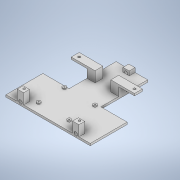
# Autodesk Inventor part: Electronics_holder
Saved by Autodesk Inventor 2020 (Build 240168000, 168)
## iProperties
Created: 2020-06-07
Part Number: Electronics_holder
Material: Generic
Document SubType Name: Modeling
Designer: Abhinav Roy
Density: 1 g/cm^3
Appearance: Default
Author: Abhinav Roy
Autodesk Inventor part; units mm, degrees
ref_plane "YZ Plane" through (0, 0, 0) normal (1, 0, 0) x (0, 1, 0)
ref_plane "XZ Plane" through (0, 0, 0) normal (0, 1, 0) x (-1, 0, 0)
ref_plane "XY Plane" through (0, 0, 0) normal (0, 0, 1) x (1, 0, 0)
sketch "Sketch1" plane through (0, 0, 0) normal (0, 1, 0) x (-1, 0, 0)
  line L0 (0, 0) -> (-30, 0)
  line L1 (-30, 0) -> (-30, -159)
  line L2 (-30, -159) -> (0, -159)
  line L3 (0, -159) -> (0, 0)
  line L4 (0, 0) -> (50, 0)
  line L5 (50, 0) -> (50, -70)
  line L6 (50, -70) -> (0, -70)
  line L7 (0, -70) -> (0, 0)
  dimension "d0" = 159
  dimension "d1" = 30
  dimension "d2" = 50
  dimension "d3" = 70
  constraints: 16 end point, 4 parallel, 2 horizontal, 2 perpendicular
  measures "d0" distance of L2.end L0.start
  measures "d1" distance of L0.start L0.end
  measures "d2" distance of L5.end L6.end
  measures "d3" distance of L4.end L5.end
extrude "Extrusion1" add sketch "Sketch1" along normal blind 4
sketch "Sketch2" plane through (0, 4, 0) normal (0, 1, 0) x (1, 0, 0)
  line L0 (-16.5, 0) -> (-16.5, 11)
  line L1 (-16.5, 11) -> (-28.5, 11)
  line L2 (30, 159) -> (0, 159) projected
  line L3 (30, 159) -> (24, 159)
  line L4 (24, 159) -> (24, 148)
  line L5 (24, 148) -> (30, 148)
  line L6 (30, 148) -> (30, 159)
  line L7 (-28.5, 11) -> (-28.5, 0)
  line L8 (-50, 0) -> (30, 0) projected
  line L9 (-16.5, 0) -> (-28.5, 0)
  line L10 (-50, 70) -> (-50, 0) projected
  line L11 (30, 0) -> (30, 159) projected
  point P0 (0, 0)
  dimension "d6" = 12
  dimension "d7" = 11
  dimension "d8" = 6
  dimension "d52" = 46.5
  constraints: 16 end point, 5 parallel, 2 perpendicular, 1 horizontal, 1 point on line, 1 vertical
  measures "d6" distance of L0.end L1.end
  measures "d7" distance of L0.start L0.end
  measures "d8" distance of L4.end L5.end
  measures "d52" distance between parallel lines of L11 L0
extrude "Extrusion2" add sketch "Sketch2" along normal blind 8 contours L6 L5 L4 L2
extrude "Extrusion4" add sketch "Sketch2" along normal blind 20 contours L8 L7 L1 L0
sketch "Sketch9" plane through (0, 4, 0) normal (0, 1, 0) x (1, 0, 0)
  line L0 (30, 0) -> (30, 148) construction
  line L1 (30, 111.5) -> (0, 111.5) construction
  line L2 (-16.5, 0) -> (30, 0) construction
  line L3 (0, 159) -> (0, 70) projected
  line L4 (15, 119) -> (0, 119)
  line L5 (0, 119) -> (0, 104) construction
  line L6 (0, 104) -> (15, 104)
  line L7 (15, 104) -> (15, 119)
  line L8 (15, 119) -> (0, 104) construction
  line L9 (0, 119) -> (15, 104) construction
  point P0 (0, 0)
  point P1 (7.5, 111.5)
  point P2 (0, 119)
  dimension "d63" = 111.5
  dimension "d64" = 15
  dimension "d65" = 15
  constraints: 14 end point, 3 point on line, 2 horizontal, 2 midpoint, 2 parallel, 1 perpendicular
  measures "d63" distance between parallel lines of L1 L2
  measures "d64" distance of L5.end L6.end
  measures "d65" distance of L6.end L4.start
extrude "Extrusion5" add sketch "Sketch9" along normal blind 20
sketch "Sketch10" plane through (0, 0, -159) normal (-1, 0, 0) x (0, 0, 1)
  line L0 (40, 24) -> (55, 24) projected
  line L1 (40, 24) -> (55, 24)
  line L2 (55, 24) -> (55, 20)
  line L3 (55, 20) -> (40, 20)
  line L4 (40, 20) -> (40, 24)
  point P0 (159, 0)
  dimension "d68" = 4
  constraints: 8 end point, 2 parallel, 1 horizontal, 1 perpendicular
  measures "d68" distance of L1.end L2.end
extrude "Extrusion6" add sketch "Sketch10" along normal blind 30
sketch "Sketch11" plane through (0, 24, 0) normal (0, 1, 0) x (1, 0, 0)
  line L0 (-30, 104) -> (-30, 119) projected
  line L1 (15, 104) -> (-30, 104) projected
  point P0 (0, 0)
  point P1 (-22.5, 111.5)
  dimension "d71" = 7.5
  dimension "d82" = 7.5
  measures "d71" distance from line of L0 point (-22.5, 111.5)
  measures "d82" distance from line of L1 point (-22.5, 111.5)
hole "Hole5" at (-22.5, 24, -111.5) direction (0, -1, 0) diameter 4.6 depth 6
mirror "Mirror1" about plane through (30, 0, 0) normal (1, 0, 0) of "Extrusion1", "Extrusion2", "Extrusion4", "Extrusion5", "Hole5", "Extrusion6"
sketch "Sketch5" plane through (0, 4, 0) normal (0, 1, 0) x (1, 0, 0)
  line L0 (-50, 0) -> (110, 0) construction
  line L1 (30, 0) -> (30, 159)
  line L2 (0, 159) -> (60, 159) projected
  line L3 (-5.5, 66.5) -> (52.5, 66.5) construction
  line L4 (52.5, 66.5) -> (52.5, 17.5) construction
  line L5 (52.5, 17.5) -> (-5.5, 17.5) construction
  line L6 (-5.5, 17.5) -> (-5.5, 66.5) construction
  line L7 (-5.5, 66.5) -> (52.5, 17.5) construction
  line L8 (52.5, 66.5) -> (-5.5, 17.5) construction
  circle A0 centre (52.5, 17.5) radius 3.5
  circle A1 centre (-5.5, 17.5) radius 3.5
  circle A2 centre (-5.5, 66.5) radius 3.5
  circle A3 centre (52.5, 66.5) radius 3.5
  point P0 (-13, 0)
  point P1 (73, 0)
  point P2 (23.5, 42)
  dimension "d31" = 58
  dimension "d32" = 49
  dimension "d33" = 7
  dimension "d45" = 42
  dimension "d79" = 13
  constraints: 14 end point, 4 centre point, 4 coincident, 4 midpoint, 3 equal radius, 2 parallel, 1 horizontal, 1 perpendicular
  measures "d31" distance of L4.end L5.end
  measures "d32" distance of L3.end L4.end
  measures "d33" diameter of A0
  measures "d45" distance from line of L0 point (23.5, 42)
  measures "d79" diameter of point (23.5, 42) L1
extrude "Extrusion3" add sketch "Sketch5" along normal blind 2
sketch "Sketch6" plane through (52.5, 6, -17.5) normal (0, 1, 0) x (1, 0, 0)
  circle A0 centre (-58, 0) radius 3.5 construction
  circle A1 centre (-58, 49) radius 3.5 construction
  circle A2 centre (0, 49) radius 3.5 construction
  point P0 (-52.5, -17.5)
  point P1 (0, 0)
  point P2 (-58, 0)
  point P3 (-58, 49)
  constraints: 3 coincident
hole "Hole3" at (52.5, 6, -66.5) at (52.5, 6, -17.5) at (-5.5, 6, -17.5) at (-5.5, 6, -66.5) direction (0, -1, 0) diameter 1.8 depth 6
sketch "Sketch4" plane through (-50, 12, 0) normal (0, 0, 1) x (1, 0, 0)
  line L0 (0, -12) -> (0, -8) projected
  line L1 (0, -12) -> (160, -12) projected
  line L2 (160, -12) -> (160, -8) projected
  line L3 (21.5, -8) -> (21.5, 12) projected
  line L4 (126.5, -8) -> (126.5, 12) projected
  point P0 (50, -12)
  point P1 (27.5, -6)
  point P2 (132.5, -6)
  point P3 (160, 0)
  dimension "d21" = 6
  dimension "d22" = 6
  dimension "d53" = 6
  dimension "d54" = 6
  measures "d21" distance from line of L1 point (27.5, -6)
  measures "d22" distance from line of L1 point (132.5, -6)
  measures "d53" distance from line of L3 point (27.5, -6)
  measures "d54" distance from line of L4 point (132.5, -6)
hole "Hole2" at (-22.5, 6, 0) at (82.5, 6, 0) direction (0, 0, -1) diameter 5.9 depth 11 countersink diameter 6.8 countersink angle 45
sketch "Sketch3" plane through (0, 0, -159) normal (0, 0, -1) x (-1, 0, 0)
  line L0 (-24, 12) -> (-36, 12) projected
  line L1 (-36, 4) -> (-36, 12) projected
  point P0 (0, 0)
  point P1 (-30, 6)
  dimension "d11" = 6
  dimension "d12" = 6
  measures "d11" distance from line of L0 point (-30, 6)
  measures "d12" distance from line of point (-30, 6) L1
hole "Hole1" at (30, 6, -159) direction (0, 0, 1) diameter 5.9 depth 11 countersink diameter 6.5 countersink angle 45
sketch "Sketch7" plane through (0, 24, 0) normal (0, 1, 0) x (1, 0, 0)
  line L0 (-16.5, 11) -> (-28.5, 11) construction
  line L1 (-28.5, 11) -> (-28.5, 0) construction
  line L2 (76.5, 11) -> (88.5, 11) construction
  line L3 (76.5, 0) -> (76.5, 11) construction
  line L4 (88.5, 0) -> (76.5, 0) projected
  line L5 (-28.5, 0) -> (-16.5, 0) projected
  point P0 (0, 0)
  point P1 (-22.5, 7)
  point P2 (82.5, 7)
  dimension "d80" = 7
  dimension "d81" = 7
  measures "d80" distance from line of L4 point (82.5, 7)
  measures "d81" distance from line of L5 point (-22.5, 7)
hole "Hole4" at (-22.5, 24, -7) at (82.5, 24, -7) direction (0, -1, 0) diameter 4.1 depth 6
body "Solid1"
